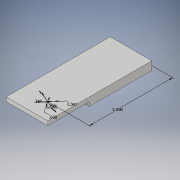
# Autodesk Inventor part: target
Saved by Autodesk Inventor 2017 (Build 210142000, 142)
## iProperties
Created: 2016-11-15
Part Number: target
Material: Generic
Document SubType Name: Modeling
Designer: Darien Morrow
Density: 1 g/cm^3
Appearance: Default
Author: Darien Morrow
Autodesk Inventor part; units mm, degrees
ref_plane "YZ Plane" through (0, 0, 0) normal (1, 0, 0) x (0, 1, 0)
ref_plane "XZ Plane" through (0, 0, 0) normal (0, 1, 0) x (-1, 0, 0)
ref_plane "XY Plane" through (0, 0, 0) normal (0, 0, 1) x (1, 0, 0)
sketch "Sketch1" plane through (0, 0, 0) normal (0, 0, 1) x (1, 0, 0)
  line L0 (-31.75, -6.35) -> (31.75, -6.35)
  line L1 (31.75, -6.35) -> (31.75, 6.35)
  line L2 (31.75, 6.35) -> (-31.75, 6.35)
  line L3 (-31.75, 6.35) -> (-31.75, -6.35)
  line L4 (-31.75, -6.35) -> (31.75, 6.35) construction
  line L5 (31.75, -6.35) -> (-31.75, 6.35) construction
  point P0 (0, 0)
  dimension "d0" = 63.5
  dimension "d1" = 12.7
  constraints: 12 end point, 2 midpoint, 2 parallel, 1 horizontal, 1 perpendicular
  measures "d0" distance between parallel lines of L1 L3
  measures "d1" distance between parallel lines of L0 L2
extrude "Extrusion1" add sketch "Sketch1" along normal blind 158.75
sketch "Sketch2" plane through (-31.75, -6.35, 0) normal (0, -1, 0) x (1, 0, 0)
  line L0 (63.5, 0) -> (63.5, 158.75) projected
  line L1 (0, 95.25) -> (63.5, 95.25)
  line L2 (63.5, 95.25) -> (63.5, 158.75)
  line L3 (63.5, 158.75) -> (0, 158.75)
  line L4 (0, 158.75) -> (0, 95.25)
  line L5 (0, 95.25) -> (63.5, 158.75) construction
  line L6 (63.5, 95.25) -> (0, 158.75) construction
  point P0 (31.75, 0)
  point P1 (31.75, 127)
  dimension "d4" = 127
  constraints: 12 end point, 2 midpoint, 2 parallel, 1 horizontal, 1 perpendicular
  measures "d4" distance of point (31.75, 0) point (31.75, 127)
extrude "Extrusion2" cut sketch "Sketch2" against normal blind 6.35
sketch "Sketch3" plane through (0, 0, 0) normal (0, 0, -1) x (-1, 0, 0)
  line L0 (31.75, 0) -> (-31.75, 0) projected
  point P0 (0, 0)
  point P1 (-25.4, 0)
  point P2 (25.4, 0)
  dimension "d7" = 25.4
  dimension "d8" = 25.4
  constraints: 1 point on line
  measures "d7" distance of point (-25.4, 0) point (0, 0)
  measures "d8" distance of point (25.4, 0) point (0, 0)
hole "Hole1" at (25.4, 0, 0) at (-25.4, 0, 0) direction (0, 0, 1) diameter 5.1054 depth 12.7 tip angle 118
sketch "Sketch4" plane through (-31.75, 0, 0) normal (0, -1, 0) x (1, 0, 0)
  line L0 (0, 0) -> (63.5, 0) projected
  circle A0 centre (31.75, 127) radius 4.4336
  circle A1 centre (31.75, 127) radius 8.8671
  circle A2 centre (31.75, 127) radius 13.2969
  circle A3 centre (31.75, 127) radius 17.7292
  circle A4 centre (31.75, 127) radius 22.1615
  point P0 (31.75, 0)
  dimension "d16" = 127
  dimension "d17" = 8.8671
  dimension "d18" = 17.7343
  dimension "d19" = 26.5938
  dimension "d20" = 35.4584
  dimension "d21" = 44.323
  constraints: 5 centre point, 5 coincident
  measures "d16" distance from line of L0 point (31.75, 127)
  measures "d17" diameter of A0
  measures "d18" diameter of A1
  measures "d19" diameter of A2
  measures "d20" diameter of A3
  measures "d21" diameter of A4
body "Solid1"
